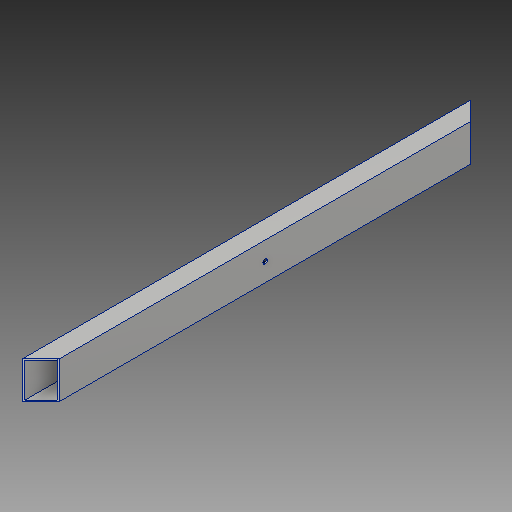
# Autodesk Inventor part: FRA_BackMainRail_002
Saved by Autodesk Inventor 2018 (Build 220112000, 112)
## iProperties
Created: 2020-01-08
Part Number: FRA_BackMainRail_002
Material: Aluminum 6061
Document SubType Name: Modeling
Designer: user
Density: 2.7 g/cm^3
Appearance: Aluminum - Flat
Mass: 369.247 g
Surface Area: 1730.29 cm^2
Volume: 136.758 cm^3
Author: user
Autodesk Inventor part; units mm, degrees
ref_plane "YZ Plane" through (0, 0, 0) normal (1, 0, 0) x (0, 1, 0)
ref_plane "XZ Plane" through (0, 0, 0) normal (0, 1, 0) x (-1, 0, 0)
ref_plane "XY Plane" through (0, 0, 0) normal (0, 0, 1) x (1, 0, 0)
sketch "Sketch1" plane through (0, 0, 0) normal (0, 0, 1) x (1, 0, 0)
  line L0 (0, 0) -> (25.4, 0)
  line L1 (25.4, 0) -> (25.4, 50.8)
  line L2 (25.4, 50.8) -> (0, 50.8)
  line L3 (0, 50.8) -> (0, 0)
  line L4 (1.5875, 1.5875) -> (23.8125, 1.5875)
  line L5 (23.8125, 1.5875) -> (23.8125, 49.2125)
  line L6 (23.8125, 49.2125) -> (1.5875, 49.2125)
  line L7 (1.5875, 49.2125) -> (1.5875, 1.5875)
  dimension "d0" = 25.4
  dimension "d1" = 50.8
  dimension "d2" = 1.5875
  constraints: 16 end point, 4 parallel, 2 perpendicular, 1 horizontal, 3 other
  measures "d0" distance of L2.end L1.end
  measures "d1" distance of L1.end L0.end
  measures "d2" distance between parallel lines of L3 L7
extrude "Extrusion1" add sketch "Sketch1" along normal mid plane 615.95
chamfer "Chamfer1" distance 25.4 angle 45 2 edges at (25.4, 25.4, 307.975) (25.4, 25.4, -307.975)
sketch "Sketch2" plane through (0, 0, 307.975) normal (-1, 0, 0) x (0, 0, 1)
  line L0 (-615.95, 0) -> (-615.95, 50.8) projected
  point P0 (-307.975, 0)
  point P1 (-307.975, 25.4)
  dimension "d8" = 25.4
  dimension "d9" = 307.975
  measures "d8" distance of point (-307.975, 0) point (-307.975, 25.4)
  measures "d9" distance from line of L0 point (-307.975, 25.4)
hole "Hole1" at (0, 25.4, 0) direction (1, 0, 0) diameter 6.35 depth 25.4 tip angle 118 counterbore diameter 9.525 counterbore depth 6.35
body "Solid1"
